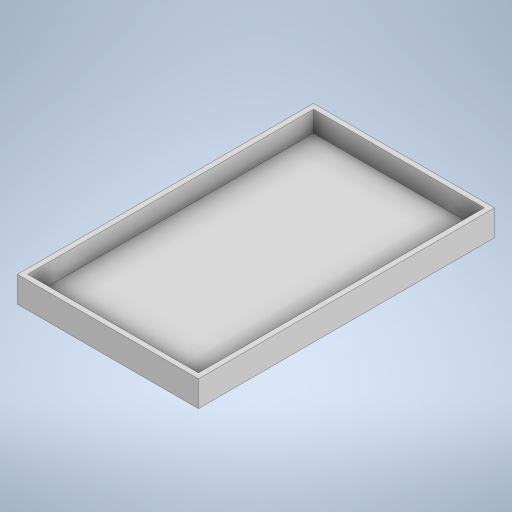
# Autodesk Inventor part: cap
Saved by Autodesk Inventor 2023 (Build 270158000, 158)
## iProperties
Created: 2023-09-17
Part Number: cap
Material: 一般
Document SubType Name: Modeling
Designer: 310611102
Density: 1 g/cm^3
Appearance: 預設
Author: 310611102
Autodesk Inventor part; units mm, degrees
ref_plane "YZ Plane" through (0, 0, 0) normal (1, 0, 0) x (0, 1, 0)
ref_plane "XZ Plane" through (0, 0, 0) normal (0, 1, 0) x (-1, 0, 0)
ref_plane "XY Plane" through (0, 0, 0) normal (0, 0, 1) x (1, 0, 0)
sketch "Sketch1" plane through (0, 0, 0) normal (0, 1, 0) x (-1, 0, 0)
  line L0 (35, 57.25) -> (-35, 57.25)
  line L1 (-35, 57.25) -> (-35, -57.25)
  line L2 (-35, -57.25) -> (35, -57.25)
  line L3 (35, -57.25) -> (35, 57.25)
  line L4 (35, 57.25) -> (-35, -57.25) construction
  line L5 (-35, 57.25) -> (35, -57.25) construction
  point P0 (0, 0)
  dimension "d0" = 70
  dimension "d1" = 114.5
  constraints: 12 end point, 2 midpoint, 2 parallel, 1 horizontal, 1 perpendicular
  measures "d0" distance of L1.end L2.end
  measures "d1" distance of L2.end L0.start
extrude "Extrusion1" add sketch "Sketch1" along normal blind 10
shell "Shell1" thickness 2 removed faces 1 at (-11.6667, 10, -19.0833)
body "Solid1"
